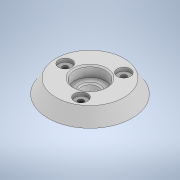
# Autodesk Inventor part: bearing_holder
Saved by Autodesk Inventor 2020 (Build 240168000, 168)
## iProperties
Created: 2019-07-23
Part Number: bearing_holder
Material: Generic
Document SubType Name: Modeling
Designer: erwin
Density: 1 g/cm^3
Appearance: Default
Author: erwin
Autodesk Inventor part; units mm, degrees
ref_plane "YZ Plane" through (0, 0, 0) normal (1, 0, 0) x (0, 1, 0)
ref_plane "XZ Plane" through (0, 0, 0) normal (0, 1, 0) x (-1, 0, 0)
ref_plane "XY Plane" through (0, 0, 0) normal (0, 0, 1) x (1, 0, 0)
sketch "Sketch1" plane through (0, 0, 0) normal (0, 1, 0) x (-1, 0, 0)
  circle A0 centre (0, 0) radius 10
  circle A1 centre (0, 0) radius 4
  dimension "d0" = 20
  dimension "d1" = 8
  constraints: 2 centre point, 2 coincident
  measures "d0" diameter of A0
  measures "d1" diameter of A1
extrude "Extrusion1" add sketch "Sketch1" along normal blind 5
sketch "Sketch2" plane through (0, 5, 0) normal (0, 1, 0) x (1, 0, 0)
  circle A0 centre (0, 0) radius 4
  circle A1 centre (0, 0) radius 30
  dimension "d4" = 8
  dimension "d5" = 60
  constraints: 2 centre point, 2 coincident
  measures "d4" diameter of A0
  measures "d5" diameter of A1
extrude "Extrusion2" add sketch "Sketch2" along normal blind 10
sketch "Sketch3" plane through (0, 15, 0) normal (0, 1, 0) x (1, 0, 0)
  circle A0 centre (0, 0) radius 11.125
  dimension "d8" = 22.25
  constraints: 1 centre point, 1 coincident
  measures "d8" diameter of A0
extrude "Extrusion3" cut sketch "Sketch3" against normal blind 7.5
draft "FaceDraft2" angle 30 pull direction (0, 1, 0) faces at (29.6115, 11.6667, 4.8123) fixed edges at (-30, 5, 0)
sketch "Sketch6" plane through (0, 15, 0) normal (0, 1, 0) x (1, 0, 0)
  line L0 (-17.6757, 0) -> (8.8379, 15.3076)
  line L1 (8.8379, 15.3076) -> (8.8379, -15.3076)
  line L2 (8.8379, -15.3076) -> (-17.6757, 0)
  circle A0 centre (0, 0) radius 11.125 construction
  line L3 (-11.125, 0) -> (-24.2265, 0) construction
  circle A1 centre (0, 0) radius 24.2265 construction
  constraints: 8 end point, 2 horizontal alignment, 1 horizontal, 1 midpoint, 2 other
hole "Hole2" at (8.8379, 15, 15.3076) at (8.8379, 15, -15.3076) at (-17.6757, 15, 0) direction (0, -1, 0) diameter 4 end through all counterbore diameter 9.5 counterbore depth 2.5
draft "FaceDraft3" angle 3 pull direction (0, -1, 0) faces at (-9.8705, 3.3333, -1.6041) fixed edges at (10, 5, 0)
sketch "Sketch7" plane through (0, 5, 0) normal (0, -1, 0) x (1, 0, 0)
  circle A0 centre (0, 0) radius 30 projected
  circle A1 centre (0, 0) radius 27
  circle A2 centre (8.8379, -15.3076) radius 2 projected
  circle A3 centre (8.8379, 15.3076) radius 2 projected
  circle A4 centre (-17.6757, 0) radius 2 projected
  circle A5 centre (0, 0) radius 30 projected
  circle A6 centre (0, 0) radius 10 projected
  dimension "d31" = 3
  constraints: 1 centre point
  measures "d31" radial gap between concentric circles of A0 A1
extrude "Extrusion5" cut sketch "Sketch7" against normal blind 0.5 contours A1
thicken "Thicken1" operation add thickness 0.5 both sides no extend neighbours yes toward (-0.9696112, -0.052336, -0.2389877) faces at (-9.6246, 3.3333, -2.3723) (9.9676, 5.3333, -0.8047)
chamfer "Chamfer1" distance 1 angle 45 1 edges at (-11.125, 15, 0)
thicken "Thicken2" operation add thickness 2 both sides no extend neighbours yes toward (-0.9870503, 0, -0.1604113) faces at (-3.9482, 4.1667, -0.6416)
chamfer "Chamfer2" distance 1 angle 45 1 edges at (-6, 7.5, 0)
chamfer "Chamfer3" distance 1 angle 45 1 edges at (10.2386, 0, 0)
body "Solid1"
